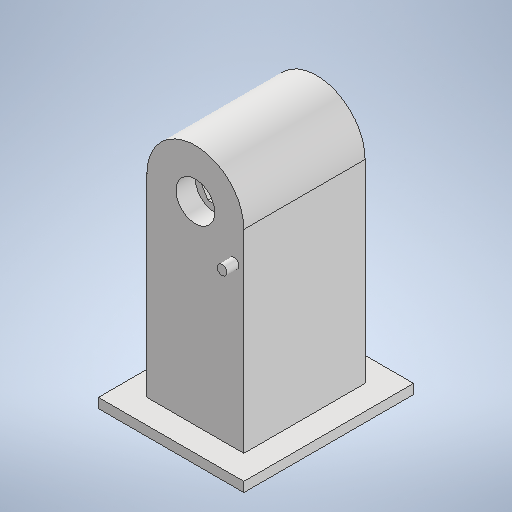
# Autodesk Inventor part: body-2
Saved by Autodesk Inventor 2025 (Build 290162000, 162)
## iProperties
Created: 2026-01-27
Part Number: body-2
Material: 一般
Document SubType Name: Modeling
Designer: mahhy
Density: 1 g/cm^3
Appearance: 既定
Author: mahhy
Autodesk Inventor part; units mm, degrees
ref_plane "YZ Plane" through (0, 0, 0) normal (1, 0, 0) x (0, 1, 0)
ref_plane "XZ Plane" through (0, 0, 0) normal (0, 1, 0) x (-1, 0, 0)
ref_plane "XY Plane" through (0, 0, 0) normal (0, 0, 1) x (1, 0, 0)
sketch "底面" plane through (0, 0, 0) normal (0, 1, 0) x (-1, 0, 0)
  line L0 (0, 0) -> (-20, 0)
  line L1 (-20, 0) -> (-20, -25)
  line L2 (-20, -25) -> (0, -25)
  line L3 (0, -25) -> (0, 0)
  dimension "d0" = 20
  dimension "d1" = 25
  constraints: 8 end point, 2 parallel, 1 horizontal, 1 perpendicular
  measures "d0" distance of L2.end L1.end
  measures "d1" distance of L1.end L0.end
extrude "本体" add sketch "底面" along normal blind 50
sketch "ねじ穴スケッチ" plane through (0, 0, 0) normal (0, 0, 1) x (1, 0, 0)
  circle A0 centre (10, 40) radius 1.45
  line L0 (0, 50) -> (20, 50) projected
  line L1 (20, 0) -> (20, 50) projected
  point P0 (0, 0)
  dimension "d6" = 10
  dimension "d9" = 2.9
  dimension "d17" = 10
  constraints: 1 centre point
  measures "d6" distance from line of L0 A0.centre
  measures "d9" diameter of A0
  measures "d17" distance from line of L1 A0.centre
extrude "ねじ穴" cut sketch "ねじ穴スケッチ" against normal blind 10
sketch "接合部スケッチ" plane through (0, 0, 0) normal (0, 0, 1) x (1, 0, 0)
  circle A0 centre (10, 40) radius 1.45 projected
  circle A1 centre (10, 40) radius 4
  point P0 (0, 0)
  dimension "d10" = 8
  constraints: 1 centre point, 1 coincident
  measures "d10" diameter of A1
extrude "接合部" cut sketch "接合部スケッチ" against normal blind 4
sketch "スケッチ4" plane through (10, 40, -4) normal (0, 0, 1) x (1, 0, 0)
  line L0 (2.875, 0) -> (1.4375, -2.4898)
  line L1 (1.4375, -2.4898) -> (-1.4375, -2.4898)
  line L2 (-1.4375, -2.4898) -> (-2.875, 0)
  line L3 (-2.875, 0) -> (-1.4375, 2.4898)
  line L4 (-1.4375, 2.4898) -> (1.4375, 2.4898)
  line L5 (1.4375, 2.4898) -> (2.875, 0)
  circle A0 centre (0, 0) radius 1.45 projected
  point P0 (-10, -40)
  point P1 (0, 2.4898)
  dimension "d13" = 2.875
  dimension "d14" = 5.75
  constraints: 12 end point, 1 coincident, 1 midpoint, 1 vertical alignment, 13 other
  measures "d13" distance of L3.end L4.end
  measures "d14" distance of L0.start L2.end
extrude "ナット穴" cut sketch "スケッチ4" against normal blind 2.4
fillet "フィレット1" radius 10 2 edges at (20, 50, -12.5) (0, 50, -12.5)
sketch "スケッチ5" plane through (0, 0, 0) normal (0, -1, 0) x (1, 0, 0)
  line L0 (25, 5) -> (-5, 5)
  line L1 (-5, 5) -> (-5, -30)
  line L2 (-5, -30) -> (25, -30)
  line L3 (25, -30) -> (25, 5)
  line L4 (0, 0) -> (20, 0) projected
  line L5 (20, 0) -> (20, -25) projected
  line L6 (0, -25) -> (0, 0) projected
  line L7 (20, -25) -> (0, -25) projected
  dimension "d19" = 5
  dimension "d20" = 5
  dimension "d21" = 5
  dimension "d22" = 5
  constraints: 8 end point, 2 parallel, 1 horizontal, 1 perpendicular
  measures "d19" distance between parallel lines of L0 L4
  measures "d20" distance between parallel lines of L5 L3
  measures "d21" distance between parallel lines of L6 L1
  measures "d22" distance between parallel lines of L7 L2
extrude "押し出し5" add sketch "スケッチ5" along normal blind 2 contours L3 L2 L1 L0 | L4 L5 L7 L6
sketch "スケッチ6" plane through (10, 40, 0) normal (0, 0, 1) x (1, 0, 0)
  circle A0 centre (8, -7) radius 1
  line L0 (15, -40) -> (-15, -40) projected
  line L1 (-10, -40) -> (-10, 0) projected
  line L2 (10, -40) -> (10, 0) projected
  dimension "d25" = 2
  dimension "d26" = 33
  dimension "d31" = 2
  constraints: 1 centre point
  measures "d25" diameter of A0
  measures "d26" distance from line of L0 A0.centre
  measures "d31" distance from line of L2 A0.centre
extrude "ストッパー" add sketch "スケッチ6" along normal blind 2.5
equation "\"d17\" = d6"
equation "\"d20\" = d19"
equation "\"d21\" = d19"
equation "\"d22\" = d19"
